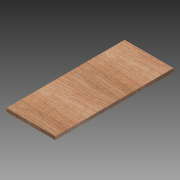
# Autodesk Inventor part: CNC-1.1v-X-5-(plate form mover for yz A)
Saved by Autodesk Inventor 2015 (Build 190159000, 159)
## iProperties
Created: 2015-07-11
Part Number: CNC-1.1v-X-5-(plate form mover for yz A)
Material: Generic
Document SubType Name: Modeling
Designer: Bangladesh
Density: 1 g/cm^3
Appearance: Default
Author: Bangladesh
Autodesk Inventor part; units mm, degrees
ref_plane "YZ Plane" through (0, 0, 0) normal (1, 0, 0) x (0, 1, 0)
ref_plane "XZ Plane" through (0, 0, 0) normal (0, 1, 0) x (-1, 0, 0)
ref_plane "XY Plane" through (0, 0, 0) normal (0, 0, 1) x (1, 0, 0)
sketch "Sketch1" plane through (0, 0, 0) normal (0, 1, 0) x (-1, 0, 0)
  line L0 (95.5, 230) -> (-95.5, 230)
  line L1 (-95.5, 230) -> (-95.5, -230)
  line L2 (-95.5, -230) -> (95.5, -230)
  line L3 (95.5, -230) -> (95.5, 230)
  line L4 (95.5, 230) -> (-95.5, -230) construction
  line L5 (-95.5, 230) -> (95.5, -230) construction
  point P0 (0, 0)
  dimension "d0" = 191
  dimension "d1" = 460
  constraints: 12 end point, 2 midpoint, 2 parallel, 1 horizontal, 1 perpendicular
  measures "d0" distance of L2.end L1.end
  measures "d1" distance of L1.end L0.end
extrude "Extrusion1" add sketch "Sketch1" along normal mid plane 13
body "Solid1"
